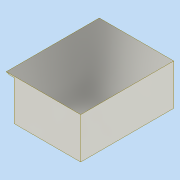
# Autodesk Inventor part: McCrea_zadne_oko_walle
Saved by Autodesk Inventor 2021 (Build 250183000, 183)
## iProperties
Created: 2022-01-17
Part Number: McCrea_zadne_oko_walle
Material: Generic
Document SubType Name: Modeling
Designer: student
Density: 1 g/cm^3
Appearance: Silver
Author: student
Autodesk Inventor part; units mm, degrees
ref_plane "YZ Plane" through (0, 0, 0) normal (1, 0, 0) x (0, 1, 0)
ref_plane "XZ Plane" through (0, 0, 0) normal (0, 1, 0) x (-1, 0, 0)
ref_plane "XY Plane" through (0, 0, 0) normal (0, 0, 1) x (1, 0, 0)
sketch "Sketch1" plane through (0, 0, 0) normal (0, 0, 1) x (1, 0, 0)
  line L0 (-23.6052, 15.8968) -> (1.3948, 15.8968)
  line L1 (1.3948, 15.8968) -> (1.3948, 0.4466)
  line L2 (1.3948, 0.4466) -> (-23.6052, 0.4466)
  line L3 (-23.6052, 0.4466) -> (-23.6052, 15.4466)
  line L4 (-23.6052, 15.8968) -> (-26.1052, 15.8968)
  line L5 (-25.6052, 15.7466) -> (-25.6052, 15.4466)
  line L6 (-25.6052, 15.4466) -> (-23.6052, 15.4466)
  line L7 (-26.1052, 15.8968) -> (-26.6052, 15.8968)
  line L8 (-26.6052, 15.8968) -> (-26.6052, 15.7466)
  line L9 (-26.6052, 15.7466) -> (-25.6052, 15.7466)
  point P0 (0, 0)
  dimension "d0" = 15
  dimension "d1" = 25
  dimension "d2" = 2
  dimension "d3" = 1
  dimension "d4" = 2.5
  dimension "d5" = 0.5
  dimension "d6" = 0.1502
  dimension "d7" = 0.3
  constraints: 20 end point, 5 perpendicular, 3 horizontal, 2 parallel
  measures "d0" distance of L2.end L3.end
  measures "d1" distance of L1.end L2.end
  measures "d2" distance of L5.end L3.end
  measures "d3" distance of L8.end L5.start
  measures "d4" distance of L0.start L4.end
  measures "d5" distance of L4.end L7.end
  measures "d6" distance of L7.end L8.end
  measures "d7" distance of L5.start L5.end
extrude "Extrusion1" add sketch "Sketch1" along normal blind 35
body "Solid1"
